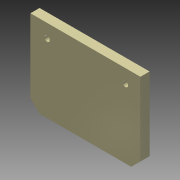
# Autodesk Inventor part: projectorMountSide_RB01
Saved by Autodesk Inventor 2013 (Build 170138000, 138)
## iProperties
Created: 2014-06-13
Part Number: projectorMountSide_RB01
Material: Nylon, molybdenum disulphide
Document SubType Name: Modeling
Designer: Byron
Density: 1.13 g/cm^3
Mass: 28.0761 g
Surface Area: 100.587 cm^2
Volume: 24.8461 cm^3
Author: Byron
Autodesk Inventor part; units mm, degrees
ref_plane "YZ Plane" through (0, 0, 0) normal (1, 0, 0) x (0, 1, 0)
ref_plane "XZ Plane" through (0, 0, 0) normal (0, 1, 0) x (-1, 0, 0)
ref_plane "XY Plane" through (0, 0, 0) normal (0, 0, 1) x (1, 0, 0)
sketch "Sketch1" plane through (0, 0, 0) normal (0, 0, 1) x (1, 0, 0)
  line L0 (-73.2051, 41.2219) -> (-136.7051, 41.2219)
  line L1 (-143.0551, 47.5719) -> (-143.0551, 98.3719)
  line L2 (-143.0551, 98.3719) -> (-66.8551, 98.3719)
  line L3 (-66.8551, 98.3719) -> (-66.8551, 47.5719)
  line L4 (-143.0551, 47.5719) -> (-136.7051, 41.2219)
  line L5 (-73.2051, 41.2219) -> (-66.8551, 47.5719)
  point P0 (0, 0)
  point P1 (-66.8551, 41.2219)
  point P2 (-143.0551, 41.2219)
  point P3 (-117.6551, 41.2219)
  point P4 (-143.0551, 66.6219)
  point P5 (-66.8551, 72.9719)
  point P6 (-92.2551, 41.2219)
  point P7 (-143.0551, 41.2219)
  point P8 (-66.8551, 41.2219)
  dimension "d0" = 76.2
  dimension "d1" = 57.15
  dimension "d10" = 6.35
  dimension "d11" = 6.35
  dimension "d12" = 6.35
  constraints: 12 end point, 11 point on line, 2 horizontal, 2 parallel, 1 midpoint, 1 perpendicular
  measures "d0" distance of L1.end L2.end
  measures "d1" distance of point (-143.055, 41.222) L1.end
  measures "d10" distance of L0.end point (-143.055, 41.222)
  measures "d11" distance of L0.start point (-66.855, 41.222)
  measures "d12" distance of L3.end point (-66.855, 41.222)
extrude "Extrusion1" add sketch "Sketch1" along normal blind 6.35
sketch "Sketch3" plane through (0, 0, 0) normal (0, 0, -1) x (-1, 0, 0)
  arc A0 (124.5928, 66.6219) -> (120.0565, 65.1716) centre (122.0928, 66.6219) ccw projected
  line L0 (124.5928, 66.6219) -> (120.0565, 65.1716) projected
  circle A1 centre (122.0928, 66.6219) radius 11
  point P0 (0, 0)
  constraints: 1 centre point, 2 other
extrude "Extrusion3" [suppressed]
sketch "Sketch4" plane through (0, 0, 0) normal (0, 0, -1) x (-1, 0, 0)
  line L0 (143.0551, 92.0219) -> (133.3409, 92.0219) construction
  line L1 (143.0551, 85.6719) -> (133.3409, 85.6719) construction
  line L2 (143.0551, 85.6719) -> (143.0551, 98.3719) construction
  line L3 (35.1051, 88.8469) -> (143.0551, 88.8469) construction
  circle A0 centre (77.2251, 88.8469) radius 1.8542
  circle A1 centre (131.4867, 88.8469) radius 1.8542
  line L4 (133.3409, 92.0219) -> (133.3409, 85.6719) projected
  point P0 (0, 0)
  dimension "d15" = 3.7084
  dimension "d16" = 3.7084
  constraints: 2 centre point, 2 end point, 1 other
  measures "d15" diameter of A0
  measures "d16" diameter of A1
extrude "Extrusion4" cut sketch "Sketch4" against normal through all
sketch "Sketch6" plane through (0, 0, 0) normal (0, 0, -1) x (-1, 0, 0)
  circle A0 centre (122.0928, 66.6219) radius 3.175 projected
  circle A1 centre (108.9583, 67.1954) radius 1.8542 projected
  circle A2 centre (122.6662, 79.7564) radius 1.8542 projected
  circle A3 centre (135.2273, 66.0485) radius 1.8542 projected
  circle A4 centre (121.5193, 53.4875) radius 1.8542 projected
  circle A5 centre (122.0928, 66.6219) radius 19.05 construction
  point P0 (0, 0)
extrude "Extrusion6" cut sketch "Sketch6" against normal through all
sketch "Sketch7" plane through (0, 0, 0) normal (0, 0, -1) x (-1, 0, 0)
  line L0 (129.6325, 92.0219) -> (129.6325, 85.6719) projected
  line L1 (79.0793, 85.6719) -> (129.6325, 85.6719) projected
  line L2 (79.0793, 85.6719) -> (79.0793, 92.0219) projected
  line L3 (79.0793, 92.0219) -> (129.6325, 92.0219) projected
  line L4 (117.0559, 92.0219) -> (91.6559, 92.0219)
  line L5 (91.6559, 92.0219) -> (91.6559, 85.6719)
  line L6 (91.6559, 85.6719) -> (117.0559, 85.6719)
  line L7 (117.0559, 85.6719) -> (117.0559, 92.0219)
  point P0 (0, 0)
  dimension "d23" = 25.4
  dimension "d24" = 12.5766
  dimension "d25" = 12.5766
  constraints: 8 end point, 2 collinear, 2 parallel, 1 horizontal, 1 perpendicular
  measures "d23" distance of L6.end L5.end
  measures "d24" distance between parallel lines of L0 L7
  measures "d25" distance between parallel lines of L2 L5
extrude "Extrusion7" cut sketch "Sketch7" against normal through all contours L7 L1 L5 L3
equation "\"d10\" = d9"
equation "\"d12\" = d11"
equation "\"d24\" = d25"
equation "\"d9\" = 6.35"
body "Solid1"
